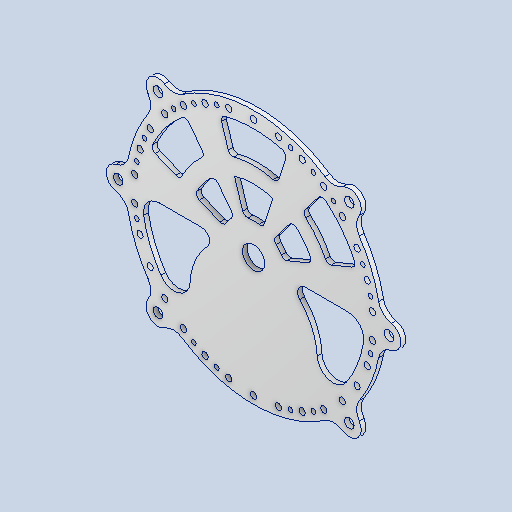
# Autodesk Inventor part: ベース板入力側
Saved by Autodesk Inventor 2024 (Build 280153000, 153)
## iProperties
Created: 2023-05-29
Part Number: ベース板入力側
Material: アルミニウム 6061
Document SubType Name: Modeling
Designer: yuta2
Density: 2.7 g/cm^3
Appearance: アルミニウム - フラット
Mass: 121.691 g
Surface Area: 362.179 cm^2
Volume: 45.0709 cm^3
Author: yuta2
Autodesk Inventor part; units mm, degrees
ref_plane "YZ Plane" through (0, 0, 0) normal (1, 0, 0) x (0, 1, 0)
ref_plane "XZ Plane" through (0, 0, 0) normal (0, 1, 0) x (-1, 0, 0)
ref_plane "XY Plane" through (0, 0, 0) normal (0, 0, 1) x (1, 0, 0)
sketch "スケッチ1" plane through (0, 0, 0) normal (0, 0, 1) x (1, 0, 0)
  circle A0 centre (0, 0) radius 80
  dimension "d0" = 160
  constraints: 1 centre point, 1 coincident
  measures "d0" diameter of A0
extrude "押し出し1" add sketch "スケッチ1" along normal blind 3
sketch "スケッチ2" plane through (0, 0, 3) normal (0, 0, 1) x (1, 0, 0)
  circle A0 centre (0, 0) radius 75
  point P0 (0, 75)
  dimension "d3" = 150
  constraints: 2 vertical alignment, 1 coincident, 2 other
hole "穴1" at (0, 75, 3) direction (0, 0, -1) diameter 4 end through all
pattern_circular "円形状パターン1" count 30 over 360 about axis through (0, 0, 0) along (0, 0, 1) of "穴1"
sketch "スケッチ3" plane through (0, 0, 3) normal (0, 0, 1) x (1, 0, 0)
  point P0 (0, 0)
  point P1 (0, 0)
  constraints: 1 coincident
hole "穴2" at (0, 0, 3) direction (0, 0, -1) diameter 14 end through all
sketch "スケッチ4" plane through (0, 0, 0) normal (0, 0, -1) x (-1, 0, 0)
  circle A0 centre (0, 0) radius 75
  line L0 (73.3611, 15.5934) -> (0, 0)
  line L1 (0, 0) -> (75, 0)
  circle A1 centre (0, 0) radius 7 projected
  line L2 (0, 0) -> (0, 75)
  line L3 (0, 0) -> (75, 0)
  point P0 (73.3611, 15.5934)
  point P1 (68.5159, 30.5052)
  point P2 (60.6763, 44.0839)
  point P3 (50.1848, 55.7359)
  point P4 (37.5, 64.9519)
  point P5 (23.1763, 71.3292)
  point P6 (-73.3611, 15.5934)
  point P7 (-68.5159, 30.5052)
  point P8 (-60.6763, 44.0839)
  point P9 (-50.1848, 55.7359)
  point P10 (-37.5, 64.9519)
  point P11 (-23.1763, 71.3292)
  point P12 (73.3611, -15.5934)
  point P13 (68.5159, -30.5052)
  point P14 (60.6763, -44.0839)
  point P15 (50.1848, -55.7359)
  point P16 (37.5, -64.9519)
  point P17 (23.1763, -71.3292)
  point P18 (-23.1763, -71.3292)
  point P19 (-37.5, -64.9519)
  point P20 (-50.1848, -55.7359)
  point P21 (-60.6763, -44.0839)
  point P22 (-68.5159, -30.5052)
  point P23 (-73.3611, -15.5934)
  dimension "d21" = 150
  dimension "d22" = 12
  dimension "d25" = 60
  constraints: 18 symmetric about line, 8 end point, 4 point on circle, 1 centre point, 1 coincident, 1 horizontal, 1 perpendicular, 1 point on line, 1 vertical, 6 other
  measures "d21" diameter of A0
  measures "d22" angle of L1 L0
hole "穴3" at (-73.3611, 15.5934, 0) at (-68.5159, 30.5052, 0) at (-50.1848, 55.7359, 0) at (-37.5, 64.9519, 0) at (-23.1763, 71.3292, 0) at (23.1763, 71.3292, 0) at (37.5, 64.9519, 0) at (50.1848, 55.7359, 0) at (68.5159, 30.5052, 0) at (73.3611, 15.5934, 0) at (-73.3611, -15.5934, 0) at (-37.5, -64.9519, 0) at (-23.1763, -71.3292, 0) at (23.1763, -71.3292, 0) at (37.5, -64.9519, 0) at (73.3611, -15.5934, 0) direction (0, 0, 1) diameter 3 end through all
thread "ねじ1" size "M3x0.5" class "6H" standard "ANSI Metric M Profile" full length
thread "ねじ2" size "M3x0.5" class "6H" standard "ANSI Metric M Profile" full length
thread "ねじ3" size "M3x0.5" class "6H" standard "ANSI Metric M Profile" full length
thread "ねじ4" size "M3x0.5" class "6H" standard "ANSI Metric M Profile" full length
thread "ねじ5" size "M3x0.5" class "6H" standard "ANSI Metric M Profile" full length
thread "ねじ6" size "M3x0.5" class "6H" standard "ANSI Metric M Profile" full length
thread "ねじ7" size "M3x0.5" class "6H" standard "ANSI Metric M Profile" full length
thread "ねじ8" size "M3x0.5" class "6H" standard "ANSI Metric M Profile" full length
thread "ねじ9" size "M3x0.5" class "6H" standard "ANSI Metric M Profile" full length
thread "ねじ10" size "M3x0.5" class "6H" standard "ANSI Metric M Profile" full length
thread "ねじ11" size "M3x0.5" class "6H" standard "ANSI Metric M Profile" full length
thread "ねじ12" size "M3x0.5" class "6H" standard "ANSI Metric M Profile" full length
thread "ねじ13" size "M3x0.5" class "6H" standard "ANSI Metric M Profile" full length
thread "ねじ14" size "M3x0.5" class "6H" standard "ANSI Metric M Profile" full length
thread "ねじ15" size "M3x0.5" class "6H" standard "ANSI Metric M Profile" full length
thread "ねじ16" size "M3x0.5" class "6H" standard "ANSI Metric M Profile" full length
sketch "スケッチ5" plane through (0, 0, 0) normal (0, 0, -1) x (-1, 0, 0)
  circle A0 centre (-85, 0) radius 7.5
  circle A1 centre (0, 0) radius 7 projected
  circle A2 centre (0, 0) radius 80 projected
  arc A3 (-86.4338, 7.3617) -> (-78.5294, 15.2686) centre (-88.3456, 17.1772) ccw
  line L0 (0, 0) -> (-62.9606, 0)
  arc A4 (-78.5294, -15.2686) -> (-86.4338, -7.3617) centre (-88.3456, -17.1772) ccw
  circle A5 centre (0, 0) radius 80 projected
  arc A6 (-66.3234, -55.9125) -> (-66.3252, -44.7321) centre (-74.6159, -50.3236) ccw
  circle A7 centre (-60.1041, -60.1041) radius 7.5
  arc A8 (-44.7321, -66.3252) -> (-55.9125, -66.3234) centre (-50.3236, -74.6159) ccw
  arc A9 (-66.3252, 44.7321) -> (-66.3234, 55.9125) centre (-74.6159, 50.3236) ccw
  circle A10 centre (-60.1041, 60.1041) radius 7.5
  arc A11 (-55.9125, 66.3234) -> (-44.7321, 66.3252) centre (-50.3236, 74.6159) ccw
  line L1 (0, 0) -> (0, 44.7321)
  point P0 (-86.4338, -7.3617)
  point P1 (-78.5294, -15.2686)
  dimension "d67" = 15
  dimension "d66" = 85
  dimension "d68" = 10
  dimension "d71" = 45
  constraints: 12 point on circle, 10 symmetric about line, 6 centre point, 4 end point, 2 horizontal, 1 horizontal alignment, 1 tangent, 1 vertical, 26 other
  measures "d66" distance of A1.centre point (-85, 0)
  measures "d68" radius of A3
extrude "押し出し2" add sketch "スケッチ5" against normal blind 3 contours A0 A2 | A3 A2 A0 | A0 A2 A4 | A9 A10 A2 | A2 A7 A6 | A10 A2 | A2 A7 | A10 A11 A2 | A2 A8 A7 picked at (-84.153, 0) picked at (-59.5052, 59.5052) picked at (-59.5052, -59.5052)
sketch "スケッチ6" plane through (0, 0, 0) normal (0, 0, -1) x (-1, 0, 0)
  arc A0 (-55.9125, 66.3234) -> (-66.3234, 55.9125) centre (-60.1041, 60.1041) ccw projected
  arc A1 (-86.4338, 7.3617) -> (-86.4338, -7.3617) centre (-85, 0) ccw projected
  arc A2 (-66.3234, -55.9125) -> (-55.9125, -66.3234) centre (-60.1041, -60.1041) ccw projected
  point P0 (0, 0)
  constraints: 3 coincident
hole "穴4" at (60.1041, 60.1041, 0) at (85, 0, 0) at (60.1041, -60.1041, 0) direction (0, 0, 1) diameter 6 end through all
pattern_circular "円形状パターン2" count 2 over 360 about axis through (0, 0, 0) along (0, 0, 1) of "押し出し2", "穴4"
sketch "スケッチ7" plane through (0, 0, 0) normal (0, 0, -1) x (-1, 0, 0)
  circle A0 centre (0, 0) radius 20
  circle A1 centre (0, 0) radius 40
  circle A2 centre (0, 0) radius 50
  circle A3 centre (0, 0) radius 70
  circle A4 centre (0, 0) radius 80
  circle A5 centre (0, 0) radius 7 projected
  line L0 (0, 0) -> (64.6716, 26.7878)
  line L1 (0, 0) -> (42.6133, 55.5347)
  line L2 (21.0494, 66.7602) -> (0, 0)
  line L3 (0, 70) -> (0, 0) construction
  line L4 (0, 0) -> (-64.6716, 26.7878)
  line L5 (0, 0) -> (-42.6133, 55.5347)
  line L6 (-21.0494, 66.7602) -> (0, 0)
  circle A6 centre (0, -36) radius 40
  circle A7 centre (0, -36) radius 30
  point P0 (-30.4381, 39.6677)
  point P1 (-46.194, 19.1342)
  point P2 (-15.0353, 47.6858)
  point P3 (15.0353, 47.6858)
  point P4 (30.4381, 39.6677)
  point P5 (46.194, 19.1342)
  point P6 (-12.1752, 15.8671)
  point P7 (-24.3505, 31.7341)
  point P8 (-36.9552, 15.3073)
  point P9 (-18.4776, 7.6537)
  point P10 (-12.0282, 38.1487)
  point P11 (-6.0141, 19.0743)
  point P12 (6.0141, 19.0743)
  point P13 (12.0282, 38.1487)
  point P14 (24.3505, 31.7341)
  point P15 (12.1752, 15.8671)
  point P16 (18.4776, 7.6537)
  point P17 (36.9552, 15.3073)
  dimension "d85" = 40
  dimension "d86" = 80
  dimension "d87" = 100
  dimension "d88" = 140
  dimension "d89" = 160
  dimension "d90" = 17.5
  dimension "d91" = 20
  dimension "d92" = 30
  dimension "d93" = 36
  dimension "d94" = 80
  dimension "d95" = 10
  constraints: 14 end point, 7 centre point, 6 coincident, 4 point on circle, 3 symmetric about line, 1 vertical, 1 vertical alignment
  measures "d85" diameter of A0
  measures "d86" diameter of A1
  measures "d87" diameter of A2
  measures "d88" diameter of A3
  measures "d89" diameter of A4
  measures "d90" angle of L2 L3
  measures "d91" angle of L2 L1
  measures "d92" angle of L1 L0
  measures "d93" distance of A6.centre point (0, 0)
  measures "d94" diameter of A6
  measures "d95" radial gap between concentric circles of A6 A7
extrude "押し出し3" cut sketch "スケッチ7" against normal blind 3 contours A0 L1 A1 L0 | A0 L6 A1 L2 | A2 L1 A3 L0 | A0 L4 A1 L5 | A2 L6 A3 L2 | A2 L4 A3 L5
sketch "スケッチ8" plane through (0, 0, 0) normal (0, 0, -1) x (-1, 0, 0)
  circle A0 centre (0, 0) radius 70
  line L0 (70, 0) -> (-70, 0)
  line L1 (-18.4776, 7.6537) -> (-36.9552, 15.3073) projected
  circle A1 centre (0, 0) radius 20
  circle A2 centre (0, -36) radius 40
  arc A3 (39.9407, -33.8222) -> (58.2468, -38.8241) centre (49.9258, -33.2778) ccw
  arc A4 (69.0209, -11.6667) -> (59.1608, 0) centre (59.1608, -10) ccw
  arc A5 (32.619, 0) -> (28.9947, -8.4444) centre (32.619, -5) ccw
  line L2 (0, 0) -> (0, -36)
  arc A6 (-58.2468, -38.8241) -> (-39.9407, -33.8222) centre (-49.9258, -33.2778) ccw
  arc A7 (-59.1608, 0) -> (-69.0209, -11.6667) centre (-59.1608, -10) ccw
  arc A8 (-28.9947, -8.4444) -> (-32.619, 0) centre (-32.619, -5) ccw
  point P0 (-28.9947, -8.4444)
  point P1 (-32.619, 0)
  point P2 (-69.0209, -11.6667)
  point P3 (-58.2468, -38.8241)
  dimension "d98" = 140
  dimension "d99" = 80
  dimension "d100" = 36
  dimension "d101" = 10
  dimension "d102" = 10
  dimension "d103" = 5
  constraints: 18 point on circle, 9 symmetric about line, 8 centre point, 6 tangent, 4 end point, 2 coincident, 2 midpoint, 2 point on line, 1 horizontal, 1 vertical, 1 vertical alignment, 6 other
  measures "d98" diameter of A0
  measures "d99" diameter of A2
  measures "d100" distance of L2.start L2.end
  measures "d101" radius of A3
  measures "d102" radius of A4
  measures "d103" radius of A5
extrude "押し出し4" cut sketch "スケッチ8" against normal blind 3 contours A0 A3 A2 A5 L0 A4 | A7 L0 A8 A2 A6 A0
fillet "フィレット1" radius 3 22 edges at (-18.4776, 7.6537, 1.5) (-12.1752, 15.8671, 1.5) (-36.9552, 15.3073, 1.5) (-24.3505, 31.7341, 1.5) (-46.194, 19.1342, 1.5) (-30.4381, 39.6677, 1.5) (-64.6716, 26.7878, 1.5) (-42.6133, 55.5347, 1.5) (-15.0353, 47.6858, 1.5) (-21.0494, 66.7602, 1.5) (21.0494, 66.7602, 1.5) (15.0353, 47.6858, 1.5) (30.4381, 39.6677, 1.5) (42.6133, 55.5347, 1.5) (64.6716, 26.7878, 1.5) (46.194, 19.1342, 1.5) (36.9552, 15.3073, 1.5) (24.3505, 31.7341, 1.5) (-6.0141, 19.0743, 1.5) (6.0141, 19.0743, 1.5) (12.1752, 15.8671, 1.5) (18.4776, 7.6537, 1.5)
equation "\"d3\" = D"
equation "\"d21\" = D"
equation "\"D\" = 150"
